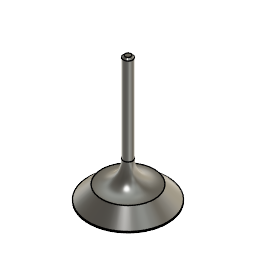
valve (Autodesk Fusion 360 design; units mm, degrees)
part number: 2026-06-07-13-37-56-352
Autodesk Fusion 360 part; units mm, degrees
sketch "Sketch1" plane through (0, 0, 0) normal (0, 1, 0) x (1, 0, 0)
sketch "Sketch2" plane through (0, 0, 0) normal (1, 0, 0) x (0, 1, 0)
sketch "Sketch3" plane through (0, 0, 0) normal (1, 0, 0) x (0, 1, 0)
  line L0 (0, 0) -> (0, 85.55)
  line L1 (0, 0) -> (26.67, 0)
  line L2 (26.67, 0) -> (26.67, 0.8152)
  line L3 (26.67, 0.8152) -> (17.7186, 9.7666)
  line L4 (0, 85.55) -> (3.18, 85.55)
  line L5 (3.18, 85.55) -> (3.18, 25)
  arc A0 (3.18, 25) -> (17.7186, 9.7666) centre (18.43, 25) ccw
  constraint coincident L0.start L1.start
  constraint vertical L0
  constraint perpendicular L0 L1
  constraint vertical L2
  constraint perpendicular L0 L4
  constraint perpendicular L4 L5
  constraint tangent L5 A0
revolve "Revolve1" add sketch "Sketch3" angle 360 about axis through (0, 0, 0) along (0, 0, 1)
chamfer "Chamfer1" distance 1.25 angle 45 1 edges at (-2.9648, 1.1499, 85.55)
